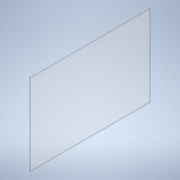
# Autodesk Inventor part: newsides
Saved by Autodesk Inventor 2020.1 (Build 241239000, 239)
## iProperties
Created: 2021-08-04
Part Number: newsides
Material: PMMA Plastic
Document SubType Name: Modeling
Designer: Caleb
Density: 1.188 g/cm^3
Appearance: Polycarbonate - Clear
Author: Caleb
Autodesk Inventor part; units mm, degrees
ref_plane "YZ Plane" through (0, 0, 0) normal (1, 0, 0) x (0, 1, 0)
ref_plane "XZ Plane" through (0, 0, 0) normal (0, 1, 0) x (-1, 0, 0)
ref_plane "XY Plane" through (0, 0, 0) normal (0, 0, 1) x (1, 0, 0)
sketch "Sketch1" plane through (0, 0, 0) normal (1, 0, 0) x (0, 1, 0)
  line L0 (-220, 325) -> (220, 325)
  line L1 (220, 325) -> (220, -325)
  line L2 (220, -325) -> (-220, -325)
  line L3 (-220, -325) -> (-220, 325)
  point P0 (0, 0)
  dimension "d4" = 440
  dimension "d5" = 650
  constraints: 8 end point, 2 parallel, 1 horizontal, 1 perpendicular
  measures "d4" distance of L0.start L0.end
  measures "d5" distance of L0.end L1.end
extrude "Extrusion1" add sketch "Sketch1" along normal mid plane 5
body "Solid1"
